Autodesk Inventor part; units mm, degrees
(part 2 of 3)
sketch "Sketch18" plane through (0, 4, 0) normal (0, 1, 0) x (1, 0, 0)
  line L0 (-39.5, -116.5) -> (-38, -116.5)
  line L1 (-38, -116.5) -> (-38, -108.5)
  line L2 (-38, -108.5) -> (-39.5, -108.5)
  line L3 (-39.5, -108.5) -> (-39.5, -116.5)
  line L4 (-40.75, -119.5) -> (-49.25, -119.5) projected
  line L5 (-40.75, -118) -> (-40.75, -119.5) projected
  line L6 (-24.5, -116.5) -> (-23, -116.5)
  line L7 (-23, -116.5) -> (-23, -108.5)
  line L8 (-23, -108.5) -> (-24.5, -108.5)
  line L9 (-24.5, -108.5) -> (-24.5, -116.5)
  line L10 (-9.5, -116.5) -> (-8, -116.5)
  line L11 (-8, -116.5) -> (-8, -108.5)
  line L12 (-8, -108.5) -> (-9.5, -108.5)
  line L13 (-9.5, -108.5) -> (-9.5, -116.5)
  line L14 (5.5, -116.5) -> (7, -116.5)
  line L15 (7, -116.5) -> (7, -108.5)
  line L16 (7, -108.5) -> (5.5, -108.5)
  line L17 (5.5, -108.5) -> (5.5, -116.5)
  line L18 (20.5, -116.5) -> (22, -116.5)
  line L19 (22, -116.5) -> (22, -108.5)
  line L20 (22, -108.5) -> (20.5, -108.5)
  line L21 (20.5, -108.5) -> (20.5, -116.5)
  line L22 (35.5, -116.5) -> (37, -116.5)
  line L23 (37, -116.5) -> (37, -108.5)
  line L24 (37, -108.5) -> (35.5, -108.5)
  line L25 (35.5, -108.5) -> (35.5, -116.5)
  line L26 (50.5, -116.5) -> (52, -116.5)
  line L27 (52, -116.5) -> (52, -108.5)
  line L28 (52, -108.5) -> (50.5, -108.5)
  line L29 (50.5, -108.5) -> (50.5, -116.5)
  line L30 (-39.5, -101.5) -> (-38, -101.5)
  line L31 (-38, -101.5) -> (-38, -93.5)
  line L32 (-38, -93.5) -> (-39.5, -93.5)
  line L33 (-39.5, -93.5) -> (-39.5, -101.5)
  line L34 (-24.5, -101.5) -> (-23, -101.5)
  line L35 (-23, -101.5) -> (-23, -93.5)
  line L36 (-23, -93.5) -> (-24.5, -93.5)
  line L37 (-24.5, -93.5) -> (-24.5, -101.5)
  line L38 (-9.5, -101.5) -> (-8, -101.5)
  line L39 (-8, -101.5) -> (-8, -93.5)
  line L40 (-8, -93.5) -> (-9.5, -93.5)
  line L41 (-9.5, -93.5) -> (-9.5, -101.5)
  line L42 (5.5, -101.5) -> (7, -101.5)
  line L43 (7, -101.5) -> (7, -93.5)
  line L44 (7, -93.5) -> (5.5, -93.5)
  line L45 (5.5, -93.5) -> (5.5, -101.5)
  line L46 (20.5, -101.5) -> (22, -101.5)
  line L47 (22, -101.5) -> (22, -93.5)
  line L48 (22, -93.5) -> (20.5, -93.5)
  line L49 (20.5, -93.5) -> (20.5, -101.5)
  line L50 (35.5, -101.5) -> (37, -101.5)
  line L51 (37, -101.5) -> (37, -93.5)
  line L52 (37, -93.5) -> (35.5, -93.5)
  line L53 (35.5, -93.5) -> (35.5, -101.5)
  line L54 (50.5, -101.5) -> (52, -101.5)
  line L55 (52, -101.5) -> (52, -93.5)
  line L56 (52, -93.5) -> (50.5, -93.5)
  line L57 (50.5, -93.5) -> (50.5, -101.5)
  line L58 (-39.5, -86.5) -> (-38, -86.5)
  line L59 (-38, -86.5) -> (-38, -78.5)
  line L60 (-38, -78.5) -> (-39.5, -78.5)
  line L61 (-39.5, -78.5) -> (-39.5, -86.5)
  line L62 (-24.5, -86.5) -> (-23, -86.5)
  line L63 (-23, -86.5) -> (-23, -78.5)
  line L64 (-23, -78.5) -> (-24.5, -78.5)
  line L65 (-24.5, -78.5) -> (-24.5, -86.5)
  line L66 (-9.5, -86.5) -> (-8, -86.5)
  line L67 (-8, -86.5) -> (-8, -78.5)
  line L68 (-8, -78.5) -> (-9.5, -78.5)
  line L69 (-9.5, -78.5) -> (-9.5, -86.5)
  line L70 (5.5, -86.5) -> (7, -86.5)
  line L71 (7, -86.5) -> (7, -78.5)
  line L72 (7, -78.5) -> (5.5, -78.5)
  line L73 (5.5, -78.5) -> (5.5, -86.5)
  line L74 (20.5, -86.5) -> (22, -86.5)
  line L75 (22, -86.5) -> (22, -78.5)
  line L76 (22, -78.5) -> (20.5, -78.5)
  line L77 (20.5, -78.5) -> (20.5, -86.5)
  line L78 (35.5, -86.5) -> (37, -86.5)
  line L79 (37, -86.5) -> (37, -78.5)
  line L80 (37, -78.5) -> (35.5, -78.5)
  line L81 (35.5, -78.5) -> (35.5, -86.5)
  line L82 (50.5, -86.5) -> (52, -86.5)
  line L83 (52, -86.5) -> (52, -78.5)
  line L84 (52, -78.5) -> (50.5, -78.5)
  line L85 (50.5, -78.5) -> (50.5, -86.5)
  line L86 (-39.5, -71.5) -> (-38, -71.5)
  line L87 (-38, -71.5) -> (-38, -63.5)
  line L88 (-38, -63.5) -> (-39.5, -63.5)
  line L89 (-39.5, -63.5) -> (-39.5, -71.5)
  line L90 (-24.5, -71.5) -> (-23, -71.5)
  line L91 (-23, -71.5) -> (-23, -63.5)
  line L92 (-23, -63.5) -> (-24.5, -63.5)
  line L93 (-24.5, -63.5) -> (-24.5, -71.5)
  line L94 (-9.5, -71.5) -> (-8, -71.5)
  line L95 (-8, -71.5) -> (-8, -63.5)
  line L96 (-8, -63.5) -> (-9.5, -63.5)
  line L97 (-9.5, -63.5) -> (-9.5, -71.5)
  line L98 (5.5, -71.5) -> (7, -71.5)
  line L99 (7, -71.5) -> (7, -63.5)
  line L100 (7, -63.5) -> (5.5, -63.5)
  line L101 (5.5, -63.5) -> (5.5, -71.5)
  line L102 (20.5, -71.5) -> (22, -71.5)
  line L103 (22, -71.5) -> (22, -63.5)
  line L104 (22, -63.5) -> (20.5, -63.5)
  line L105 (20.5, -63.5) -> (20.5, -71.5)
  line L106 (35.5, -71.5) -> (37, -71.5)
  line L107 (37, -71.5) -> (37, -63.5)
  line L108 (37, -63.5) -> (35.5, -63.5)
  line L109 (35.5, -63.5) -> (35.5, -71.5)
  line L110 (50.5, -71.5) -> (52, -71.5)
  line L111 (52, -71.5) -> (52, -63.5)
  line L112 (52, -63.5) -> (50.5, -63.5)
  line L113 (50.5, -63.5) -> (50.5, -71.5)
  line L114 (-39.5, -56.5) -> (-38, -56.5)
  line L115 (-38, -56.5) -> (-38, -48.5)
  line L116 (-38, -48.5) -> (-39.5, -48.5)
  line L117 (-39.5, -48.5) -> (-39.5, -56.5)
  line L118 (-24.5, -56.5) -> (-23, -56.5)
  line L119 (-23, -56.5) -> (-23, -48.5)
  line L120 (-23, -48.5) -> (-24.5, -48.5)
  line L121 (-24.5, -48.5) -> (-24.5, -56.5)
  line L122 (-9.5, -56.5) -> (-8, -56.5)
  line L123 (-8, -56.5) -> (-8, -48.5)
  line L124 (-8, -48.5) -> (-9.5, -48.5)
  line L125 (-9.5, -48.5) -> (-9.5, -56.5)
  line L126 (5.5, -56.5) -> (7, -56.5)
  line L127 (7, -56.5) -> (7, -48.5)
  line L128 (7, -48.5) -> (5.5, -48.5)
  line L129 (5.5, -48.5) -> (5.5, -56.5)
  line L130 (20.5, -56.5) -> (22, -56.5)
  line L131 (22, -56.5) -> (22, -48.5)
  line L132 (22, -48.5) -> (20.5, -48.5)
  line L133 (20.5, -48.5) -> (20.5, -56.5)
  line L134 (35.5, -56.5) -> (37, -56.5)
  line L135 (37, -56.5) -> (37, -48.5)
  line L136 (37, -48.5) -> (35.5, -48.5)
  line L137 (35.5, -48.5) -> (35.5, -56.5)
  line L138 (50.5, -56.5) -> (52, -56.5)
  line L139 (52, -56.5) -> (52, -48.5)
  line L140 (52, -48.5) -> (50.5, -48.5)
  line L141 (50.5, -48.5) -> (50.5, -56.5)
  line L142 (-39.5, -41.5) -> (-38, -41.5)
  line L143 (-38, -41.5) -> (-38, -33.5)
  line L144 (-38, -33.5) -> (-39.5, -33.5)
  line L145 (-39.5, -33.5) -> (-39.5, -41.5)
  line L146 (-24.5, -41.5) -> (-23, -41.5)
  line L147 (-23, -41.5) -> (-23, -33.5)
  line L148 (-23, -33.5) -> (-24.5, -33.5)
  line L149 (-24.5, -33.5) -> (-24.5, -41.5)
  line L150 (-9.5, -41.5) -> (-8, -41.5)
  line L151 (-8, -41.5) -> (-8, -33.5)
  line L152 (-8, -33.5) -> (-9.5, -33.5)
  line L153 (-9.5, -33.5) -> (-9.5, -41.5)
  line L154 (5.5, -41.5) -> (7, -41.5)
  line L155 (7, -41.5) -> (7, -33.5)
  line L156 (7, -33.5) -> (5.5, -33.5)
  line L157 (5.5, -33.5) -> (5.5, -41.5)
  line L158 (20.5, -41.5) -> (22, -41.5)
  line L159 (22, -41.5) -> (22, -33.5)
  line L160 (22, -33.5) -> (20.5, -33.5)
  line L161 (20.5, -33.5) -> (20.5, -41.5)
  line L162 (35.5, -41.5) -> (37, -41.5)
  line L163 (37, -41.5) -> (37, -33.5)
  line L164 (37, -33.5) -> (35.5, -33.5)
  line L165 (35.5, -33.5) -> (35.5, -41.5)
  line L166 (50.5, -41.5) -> (52, -41.5)
  line L167 (52, -41.5) -> (52, -33.5)
  line L168 (52, -33.5) -> (50.5, -33.5)
  line L169 (50.5, -33.5) -> (50.5, -41.5)
  line L170 (-39.5, -26.5) -> (-38, -26.5)
  line L171 (-38, -26.5) -> (-38, -18.5)
  line L172 (-38, -18.5) -> (-39.5, -18.5)
  line L173 (-39.5, -18.5) -> (-39.5, -26.5)
  line L174 (-24.5, -26.5) -> (-23, -26.5)
  line L175 (-23, -26.5) -> (-23, -18.5)
  line L176 (-23, -18.5) -> (-24.5, -18.5)
  line L177 (-24.5, -18.5) -> (-24.5, -26.5)
  line L178 (-9.5, -26.5) -> (-8, -26.5)
  line L179 (-8, -26.5) -> (-8, -18.5)
  line L180 (-8, -18.5) -> (-9.5, -18.5)
  line L181 (-9.5, -18.5) -> (-9.5, -26.5)
  line L182 (5.5, -26.5) -> (7, -26.5)
  line L183 (7, -26.5) -> (7, -18.5)
  line L184 (7, -18.5) -> (5.5, -18.5)
  line L185 (5.5, -18.5) -> (5.5, -26.5)
  line L186 (20.5, -26.5) -> (22, -26.5)
  line L187 (22, -26.5) -> (22, -18.5)
  line L188 (22, -18.5) -> (20.5, -18.5)
  line L189 (20.5, -18.5) -> (20.5, -26.5)
  line L190 (35.5, -26.5) -> (37, -26.5)
  line L191 (37, -26.5) -> (37, -18.5)
  line L192 (37, -18.5) -> (35.5, -18.5)
  line L193 (35.5, -18.5) -> (35.5, -26.5)
  line L194 (50.5, -26.5) -> (52, -26.5)
  line L195 (52, -26.5) -> (52, -18.5)
  line L196 (52, -18.5) -> (50.5, -18.5)
  line L197 (50.5, -18.5) -> (50.5, -26.5)
  line L198 (-39.5, -11.5) -> (-38, -11.5)
  line L199 (-38, -11.5) -> (-38, -3.5)
  line L200 (-38, -3.5) -> (-39.5, -3.5)
  line L201 (-39.5, -3.5) -> (-39.5, -11.5)
  line L202 (-24.5, -11.5) -> (-23, -11.5)
  line L203 (-23, -11.5) -> (-23, -3.5)
  line L204 (-23, -3.5) -> (-24.5, -3.5)
  line L205 (-24.5, -3.5) -> (-24.5, -11.5)
  line L206 (-9.5, -11.5) -> (-8, -11.5)
  line L207 (-8, -11.5) -> (-8, -3.5)
  line L208 (-8, -3.5) -> (-9.5, -3.5)
  line L209 (-9.5, -3.5) -> (-9.5, -11.5)
  line L210 (5.5, -11.5) -> (7, -11.5)
  line L211 (7, -11.5) -> (7, -3.5)
  line L212 (7, -3.5) -> (5.5, -3.5)
  line L213 (5.5, -3.5) -> (5.5, -11.5)
  line L214 (20.5, -11.5) -> (22, -11.5)
  line L215 (22, -11.5) -> (22, -3.5)
  line L216 (22, -3.5) -> (20.5, -3.5)
  line L217 (20.5, -3.5) -> (20.5, -11.5)
  line L218 (35.5, -11.5) -> (37, -11.5)
  line L219 (37, -11.5) -> (37, -3.5)
  line L220 (37, -3.5) -> (35.5, -3.5)
  line L221 (35.5, -3.5) -> (35.5, -11.5)
  line L222 (50.5, -11.5) -> (52, -11.5)
  line L223 (52, -11.5) -> (52, -3.5)
  line L224 (52, -3.5) -> (50.5, -3.5)
  line L225 (50.5, -3.5) -> (50.5, -11.5)
  line L226 (-39.5, 3.5) -> (-38, 3.5)
  line L227 (-38, 3.5) -> (-38, 11.5)
  line L228 (-38, 11.5) -> (-39.5, 11.5)
  line L229 (-39.5, 11.5) -> (-39.5, 3.5)
  line L230 (-24.5, 3.5) -> (-23, 3.5)
  line L231 (-23, 3.5) -> (-23, 11.5)
  line L232 (-23, 11.5) -> (-24.5, 11.5)
  line L233 (-24.5, 11.5) -> (-24.5, 3.5)
  line L234 (-9.5, 3.5) -> (-8, 3.5)
  line L235 (-8, 3.5) -> (-8, 11.5)
  line L236 (-8, 11.5) -> (-9.5, 11.5)
  line L237 (-9.5, 11.5) -> (-9.5, 3.5)
  line L238 (5.5, 3.5) -> (7, 3.5)
  line L239 (7, 3.5) -> (7, 11.5)
  line L240 (7, 11.5) -> (5.5, 11.5)
  line L241 (5.5, 11.5) -> (5.5, 3.5)
  line L242 (20.5, 3.5) -> (22, 3.5)
  line L243 (22, 3.5) -> (22, 11.5)
  line L244 (22, 11.5) -> (20.5, 11.5)
  line L245 (20.5, 11.5) -> (20.5, 3.5)
  line L246 (35.5, 3.5) -> (37, 3.5)
  line L247 (37, 3.5) -> (37, 11.5)
  line L248 (37, 11.5) -> (35.5, 11.5)
  line L249 (35.5, 11.5) -> (35.5, 3.5)
  line L250 (50.5, 3.5) -> (52, 3.5)
  line L251 (52, 3.5) -> (52, 11.5)
  line L252 (52, 11.5) -> (50.5, 11.5)
  line L253 (50.5, 11.5) -> (50.5, 3.5)
  line L254 (-39.5, 18.5) -> (-38, 18.5)
  line L255 (-38, 18.5) -> (-38, 26.5)
  line L256 (-38, 26.5) -> (-39.5, 26.5)
  line L257 (-39.5, 26.5) -> (-39.5, 18.5)
  line L258 (-24.5, 18.5) -> (-23, 18.5)
  line L259 (-23, 18.5) -> (-23, 26.5)
  line L260 (-23, 26.5) -> (-24.5, 26.5)
  line L261 (-24.5, 26.5) -> (-24.5, 18.5)
  line L262 (-9.5, 18.5) -> (-8, 18.5)
  line L263 (-8, 18.5) -> (-8, 26.5)
  line L264 (-8, 26.5) -> (-9.5, 26.5)
  line L265 (-9.5, 26.5) -> (-9.5, 18.5)
  line L266 (5.5, 18.5) -> (7, 18.5)
  line L267 (7, 18.5) -> (7, 26.5)
  line L268 (7, 26.5) -> (5.5, 26.5)
  line L269 (5.5, 26.5) -> (5.5, 18.5)
  line L270 (20.5, 18.5) -> (22, 18.5)
  line L271 (22, 18.5) -> (22, 26.5)
  line L272 (22, 26.5) -> (20.5, 26.5)
  line L273 (20.5, 26.5) -> (20.5, 18.5)
  line L274 (35.5, 18.5) -> (37, 18.5)
  line L275 (37, 18.5) -> (37, 26.5)
  line L276 (37, 26.5) -> (35.5, 26.5)
  line L277 (35.5, 26.5) -> (35.5, 18.5)
  line L278 (50.5, 18.5) -> (52, 18.5)
  line L279 (52, 18.5) -> (52, 26.5)
  line L280 (52, 26.5) -> (50.5, 26.5)
  line L281 (50.5, 26.5) -> (50.5, 18.5)
  line L282 (-39.5, 33.5) -> (-38, 33.5)
  line L283 (-38, 33.5) -> (-38, 41.5)
  line L284 (-38, 41.5) -> (-39.5, 41.5)
  line L285 (-39.5, 41.5) -> (-39.5, 33.5)
  line L286 (-24.5, 33.5) -> (-23, 33.5)
  line L287 (-23, 33.5) -> (-23, 41.5)
  line L288 (-23, 41.5) -> (-24.5, 41.5)
  line L289 (-24.5, 41.5) -> (-24.5, 33.5)
  line L290 (-9.5, 33.5) -> (-8, 33.5)
  line L291 (-8, 33.5) -> (-8, 41.5)
  line L292 (-8, 41.5) -> (-9.5, 41.5)
  line L293 (-9.5, 41.5) -> (-9.5, 33.5)
  line L294 (5.5, 33.5) -> (7, 33.5)
  line L295 (7, 33.5) -> (7, 41.5)
  line L296 (7, 41.5) -> (5.5, 41.5)
  line L297 (5.5, 41.5) -> (5.5, 33.5)
  line L298 (20.5, 33.5) -> (22, 33.5)
  line L299 (22, 33.5) -> (22, 41.5)
  line L300 (22, 41.5) -> (20.5, 41.5)
  line L301 (20.5, 41.5) -> (20.5, 33.5)
  line L302 (35.5, 33.5) -> (37, 33.5)
  line L303 (37, 33.5) -> (37, 41.5)
  line L304 (37, 41.5) -> (35.5, 41.5)
  line L305 (35.5, 41.5) -> (35.5, 33.5)
  line L306 (50.5, 33.5) -> (52, 33.5)
  line L307 (52, 33.5) -> (52, 41.5)
  line L308 (52, 41.5) -> (50.5, 41.5)
  line L309 (50.5, 41.5) -> (50.5, 33.5)
  line L310 (-39.5, 48.5) -> (-38, 48.5)
  line L311 (-38, 48.5) -> (-38, 56.5)
  line L312 (-38, 56.5) -> (-39.5, 56.5)
  line L313 (-39.5, 56.5) -> (-39.5, 48.5)
  line L314 (-24.5, 48.5) -> (-23, 48.5)
  line L315 (-23, 48.5) -> (-23, 56.5)
  line L316 (-23, 56.5) -> (-24.5, 56.5)
  line L317 (-24.5, 56.5) -> (-24.5, 48.5)
  line L318 (-9.5, 48.5) -> (-8, 48.5)
  line L319 (-8, 48.5) -> (-8, 56.5)
  line L320 (-8, 56.5) -> (-9.5, 56.5)
  line L321 (-9.5, 56.5) -> (-9.5, 48.5)
  line L322 (5.5, 48.5) -> (7, 48.5)
  line L323 (7, 48.5) -> (7, 56.5)
  line L324 (7, 56.5) -> (5.5, 56.5)
  line L325 (5.5, 56.5) -> (5.5, 48.5)
  line L326 (20.5, 48.5) -> (22, 48.5)
  line L327 (22, 48.5) -> (22, 56.5)
  line L328 (22, 56.5) -> (20.5, 56.5)
  line L329 (20.5, 56.5) -> (20.5, 48.5)
  line L330 (35.5, 48.5) -> (37, 48.5)
  line L331 (37, 48.5) -> (37, 56.5)
  line L332 (37, 56.5) -> (35.5, 56.5)
  line L333 (35.5, 56.5) -> (35.5, 48.5)
  line L334 (50.5, 48.5) -> (52, 48.5)
  line L335 (52, 48.5) -> (52, 56.5)
  line L336 (52, 56.5) -> (50.5, 56.5)
  line L337 (50.5, 56.5) -> (50.5, 48.5)
  line L338 (-39.5, 63.5) -> (-38, 63.5)
  line L339 (-38, 63.5) -> (-38, 71.5)
  line L340 (-38, 71.5) -> (-39.5, 71.5)
  line L341 (-39.5, 71.5) -> (-39.5, 63.5)
  line L342 (-24.5, 63.5) -> (-23, 63.5)
  line L343 (-23, 63.5) -> (-23, 71.5)
  line L344 (-23, 71.5) -> (-24.5, 71.5)
  line L345 (-24.5, 71.5) -> (-24.5, 63.5)
  line L346 (-9.5, 63.5) -> (-8, 63.5)
  line L347 (-8, 63.5) -> (-8, 71.5)
  line L348 (-8, 71.5) -> (-9.5, 71.5)
  line L349 (-9.5, 71.5) -> (-9.5, 63.5)
  line L350 (5.5, 63.5) -> (7, 63.5)
  line L351 (7, 63.5) -> (7, 71.5)
  line L352 (7, 71.5) -> (5.5, 71.5)
  line L353 (5.5, 71.5) -> (5.5, 63.5)
  line L354 (20.5, 63.5) -> (22, 63.5)
  line L355 (22, 63.5) -> (22, 71.5)
  line L356 (22, 71.5) -> (20.5, 71.5)
  line L357 (20.5, 71.5) -> (20.5, 63.5)
  line L358 (35.5, 63.5) -> (37, 63.5)
  line L359 (37, 63.5) -> (37, 71.5)
  line L360 (37, 71.5) -> (35.5, 71.5)
  line L361 (35.5, 71.5) -> (35.5, 63.5)
  line L362 (50.5, 63.5) -> (52, 63.5)
  line L363 (52, 63.5) -> (52, 71.5)
  line L364 (52, 71.5) -> (50.5, 71.5)
  line L365 (50.5, 71.5) -> (50.5, 63.5)
  line L366 (-39.5, 78.5) -> (-38, 78.5)
  line L367 (-38, 78.5) -> (-38, 86.5)
  line L368 (-38, 86.5) -> (-39.5, 86.5)
  line L369 (-39.5, 86.5) -> (-39.5, 78.5)
  line L370 (-24.5, 78.5) -> (-23, 78.5)
  line L371 (-23, 78.5) -> (-23, 86.5)
  line L372 (-23, 86.5) -> (-24.5, 86.5)
  line L373 (-24.5, 86.5) -> (-24.5, 78.5)
  line L374 (-9.5, 78.5) -> (-8, 78.5)
  line L375 (-8, 78.5) -> (-8, 86.5)
  line L376 (-8, 86.5) -> (-9.5, 86.5)
  line L377 (-9.5, 86.5) -> (-9.5, 78.5)
  line L378 (5.5, 78.5) -> (7, 78.5)
  line L379 (7, 78.5) -> (7, 86.5)
  line L380 (7, 86.5) -> (5.5, 86.5)
  line L381 (5.5, 86.5) -> (5.5, 78.5)
  line L382 (20.5, 78.5) -> (22, 78.5)
  line L383 (22, 78.5) -> (22, 86.5)
  line L384 (22, 86.5) -> (20.5, 86.5)
  line L385 (20.5, 86.5) -> (20.5, 78.5)
  line L386 (35.5, 78.5) -> (37, 78.5)
  line L387 (37, 78.5) -> (37, 86.5)
  line L388 (37, 86.5) -> (35.5, 86.5)
  line L389 (35.5, 86.5) -> (35.5, 78.5)
  line L390 (50.5, 78.5) -> (52, 78.5)
  line L391 (52, 78.5) -> (52, 86.5)
  line L392 (52, 86.5) -> (50.5, 86.5)
  line L393 (50.5, 86.5) -> (50.5, 78.5)
  line L394 (-39.5, 93.5) -> (-38, 93.5)
  line L395 (-38, 93.5) -> (-38, 101.5)
  line L396 (-38, 101.5) -> (-39.5, 101.5)
  line L397 (-39.5, 101.5) -> (-39.5, 93.5)
  line L398 (-24.5, 93.5) -> (-23, 93.5)
  line L399 (-23, 93.5) -> (-23, 101.5)
  line L400 (-23, 101.5) -> (-24.5, 101.5)
  line L401 (-24.5, 101.5) -> (-24.5, 93.5)
  line L402 (-9.5, 93.5) -> (-8, 93.5)
  line L403 (-8, 93.5) -> (-8, 101.5)
  line L404 (-8, 101.5) -> (-9.5, 101.5)
  line L405 (-9.5, 101.5) -> (-9.5, 93.5)
  line L406 (5.5, 93.5) -> (7, 93.5)
  line L407 (7, 93.5) -> (7, 101.5)
  line L408 (7, 101.5) -> (5.5, 101.5)
  line L409 (5.5, 101.5) -> (5.5, 93.5)
  line L410 (20.5, 93.5) -> (22, 93.5)
  line L411 (22, 93.5) -> (22, 101.5)
  line L412 (22, 101.5) -> (20.5, 101.5)
  line L413 (20.5, 101.5) -> (20.5, 93.5)
  line L414 (35.5, 93.5) -> (37, 93.5)
  line L415 (37, 93.5) -> (37, 101.5)
  line L416 (37, 101.5) -> (35.5, 101.5)
  line L417 (35.5, 101.5) -> (35.5, 93.5)
  line L418 (50.5, 93.5) -> (52, 93.5)
  line L419 (52, 93.5) -> (52, 101.5)
  line L420 (52, 101.5) -> (50.5, 101.5)
  line L421 (50.5, 101.5) -> (50.5, 93.5)
  line L422 (-39.5, 108.5) -> (-38, 108.5)
  line L423 (-38, 108.5) -> (-38, 116.5)
  line L424 (-38, 116.5) -> (-39.5, 116.5)
  line L425 (-39.5, 116.5) -> (-39.5, 108.5)
  line L426 (-24.5, 108.5) -> (-23, 108.5)
  line L427 (-23, 108.5) -> (-23, 116.5)
  line L428 (-23, 116.5) -> (-24.5, 116.5)
  line L429 (-24.5, 116.5) -> (-24.5, 108.5)
  line L430 (-9.5, 108.5) -> (-8, 108.5)
  line L431 (-8, 108.5) -> (-8, 116.5)
  line L432 (-8, 116.5) -> (-9.5, 116.5)
  line L433 (-9.5, 116.5) -> (-9.5, 108.5)
  line L434 (5.5, 108.5) -> (7, 108.5)
  line L435 (7, 108.5) -> (7, 116.5)
  line L436 (7, 116.5) -> (5.5, 116.5)
  line L437 (5.5, 116.5) -> (5.5, 108.5)
  line L438 (20.5, 108.5) -> (22, 108.5)
  line L439 (22, 108.5) -> (22, 116.5)
  line L440 (22, 116.5) -> (20.5, 116.5)
  line L441 (20.5, 116.5) -> (20.5, 108.5)
  line L442 (35.5, 108.5) -> (37, 108.5)
  line L443 (37, 108.5) -> (37, 116.5)
  line L444 (37, 116.5) -> (35.5, 116.5)
  line L445 (35.5, 116.5) -> (35.5, 108.5)
  line L446 (50.5, 108.5) -> (52, 108.5)
  line L447 (52, 108.5) -> (52, 116.5)
  line L448 (52, 116.5) -> (50.5, 116.5)
  line L449 (50.5, 116.5) -> (50.5, 108.5)
  line L450 (19.25, -89.5) -> (10.75, -89.5) projected
  line L451 (20.5, -82.75) -> (22, -82.75)
  line L452 (22, -82.75) -> (22, -74.75)
  line L453 (22, -74.75) -> (20.5, -74.75)
  line L454 (20.5, -74.75) -> (20.5, -82.75)
  line L455 (20.5, -60.25) -> (22, -60.25)
  line L456 (22, -60.25) -> (22, -52.25)
  line L457 (22, -52.25) -> (20.5, -52.25)
  line L458 (20.5, -52.25) -> (20.5, -60.25)
  line L459 (20.5, -37.75) -> (22, -37.75)
  line L460 (22, -37.75) -> (22, -29.75)
  line L461 (22, -29.75) -> (20.5, -29.75)
  line L462 (20.5, -29.75) -> (20.5, -37.75)
  line L463 (19.25, -44.5) -> (10.75, -44.5) projected
  line L464 (20.5, -19) -> (22, -19)
  line L465 (22, -19) -> (22, -11)
  line L466 (22, -11) -> (20.5, -11)
  line L467 (20.5, -11) -> (20.5, -19)
  line L468 (10.75, -20.5) -> (19.25, -20.5) projected
  line L469 (19.25, -22) -> (10.75, -22) projected
  line L470 (19.25, -8) -> (19.25, -9.5) projected
  line L471 (20.5, -0.25) -> (22, -0.25)
  line L472 (22, -0.25) -> (22, 7.75)
  line L473 (22, 7.75) -> (20.5, 7.75)
  line L474 (20.5, 7.75) -> (20.5, -0.25)
  line L475 (20.5, 22.25) -> (22, 22.25)
  line L476 (22, 22.25) -> (22, 30.25)
  line L477 (22, 30.25) -> (20.5, 30.25)
  line L478 (20.5, 30.25) -> (20.5, 22.25)
  line L479 (20.5, 44.75) -> (22, 44.75)
  line L480 (22, 44.75) -> (22, 52.75)
  line L481 (22, 52.75) -> (20.5, 52.75)
  line L482 (20.5, 52.75) -> (20.5, 44.75)
  line L483 (20.5, 67.25) -> (22, 67.25)
  line L484 (22, 67.25) -> (22, 75.25)
  line L485 (22, 75.25) -> (20.5, 75.25)
  line L486 (20.5, 75.25) -> (20.5, 67.25)
  line L487 (20.5, 86) -> (22, 86)
  line L488 (22, 86) -> (22, 94)
  line L489 (22, 94) -> (20.5, 94)
  line L490 (20.5, 94) -> (20.5, 86)
  line L491 (20.5, 104.75) -> (22, 104.75)
  line L492 (22, 104.75) -> (22, 112.75)
  line L493 (22, 112.75) -> (20.5, 112.75)
  line L494 (20.5, 112.75) -> (20.5, 104.75)
  line L495 (19.25, 83) -> (10.75, 83) projected
  line L496 (19.25, 60.5) -> (10.75, 60.5) projected
  line L497 (10.75, 59.5) -> (19.25, 59.5) projected
  line L498 (10.75, 14.5) -> (19.25, 14.5) projected
  line L499 (10.75, -45.5) -> (19.25, -45.5) projected
  line L500 (19.25, 98) -> (10.75, 98) projected
  line L501 (10.75, 37) -> (19.25, 37) projected
  point P0 (0, 0)
  point P1 (20.5, -81.75)
  point P2 (20.5, -63)
  point P3 (22, -55)
  point P4 (20.5, -36.25)
  point P5 (20.5, -21.75)
  point P6 (20.25, -7)
  point P7 (20.5, 8.75)
  point P8 (22, 0.75)
  point P9 (20.5, 23.25)
  point P10 (22, 31.25)
  point P11 (20.5, 42)
  point P12 (22, 50)
  point P13 (20.5, 68.75)
  point P14 (22, 60.75)
  point P15 (20.5, 83.25)
  point P16 (22, 113.75)
  point P17 (20.5, 112.75)
  point P18 (20.5, 108.5)
  point P19 (22, 108.5)
  point P20 (20.5, 86)
  point P21 (22, 86)
  point P22 (22, 86.5)
  point P23 (22, 93.5)
  point P24 (22, 94)
  point P25 (20.5, 94)
  point P26 (20.5, 93.5)
  point P27 (20.5, 86.5)
  point P28 (22, 67.25)
  point P29 (22, 71.5)
  point P30 (20.5, 71.5)
  point P31 (20.5, 52.75)
  point P32 (20.5, 48.5)
  point P33 (22, 48.5)
  point P34 (22, 22.25)
  point P35 (22, 26.5)
  point P36 (20.5, 26.5)
  point P37 (20.5, 7.75)
  point P38 (20.5, 3.5)
  point P39 (22, 3.5)
  point P40 (20.5, -19)
  point P41 (22, -19)
  point P42 (22, -18.5)
  point P43 (22, -11.5)
  point P44 (22, -11)
  point P45 (20.5, -11)
  point P46 (20.5, -11.5)
  point P47 (20.5, -18.5)
  point P48 (22, -37.75)
  point P49 (22, -33.5)
  point P50 (20.5, -33.5)
  point P51 (20.5, -52.25)
  point P52 (20.5, -56.5)
  point P53 (22, -56.5)
  point P54 (22, -82.75)
  point P55 (22, -78.5)
  point P56 (20.5, -78.5)
  dimension "d177" = 8
  dimension "d178" = 1.5
  dimension "d179" = 3
  dimension "d180" = 1.25
  dimension "d187" = 15
  dimension "d190" = 15
  dimension "d296" = 6.75
  dimension "d297" = 8
  dimension "d298" = 1.5
  dimension "d300" = 8
  dimension "d301" = 6.75
  dimension "d302" = 8
  dimension "d303" = 1.5
  dimension "d304" = 8
  dimension "d306" = 3
  dimension "d307" = 1.5
  dimension "d308" = 1.25
  dimension "d309" = 8
  dimension "d310" = 8
  dimension "d311" = 8
  dimension "d312" = 8
  dimension "d313" = 8
  dimension "d314" = 8
  dimension "d316" = 3
  dimension "d317" = 6.75
  dimension "d318" = 6.75
  dimension "d320" = 6.75
  dimension "d321" = 1.5
  dimension "d323" = 6.75
  dimension "d324" = 6.75
  dimension "d325" = 6.75
  constraints: 976 end point, 30 point on line, 22 parallel, 12 horizontal, 11 perpendicular, 1 vertical, 889 other
  measures "d177" distance of L2.end L0.start
  measures "d178" distance of L1.end L2.end
  measures "d179" distance between parallel lines of L4 L0
  measures "d180" distance between parallel lines of L5 L3
  measures "d187" distance of L0.start L6.start
  measures "d190" distance of L0.start L30.start
  measures "d296" distance between parallel lines of L450 L451
  measures "d297" distance of L451.end L452.end
  measures "d298" distance of L452.end L453.end
  measures "d300" distance of L455.end L456.end
  measures "d301" distance between parallel lines of L463 L459
  measures "d302" distance of L459.end L460.end
  measures "d303" distance of L460.end L461.end
  measures "d304" distance of L464.end L465.end
  measures "d306" distance between parallel lines of L469 L464
  measures "d307" distance of L465.end L466.end
  measures "d309" distance of L471.end L472.end
  measures "d310" distance of L475.end L476.end
  measures "d311" distance of L479.end L480.end
  measures "d312" distance of L483.end L484.end
  measures "d313" distance of L487.end L488.end
  measures "d314" distance of L491.end L492.end
  measures "d316" distance between parallel lines of L495 L487
  measures "d317" distance between parallel lines of L496 L483
  measures "d318" distance between parallel lines of L497 L481
  measures "d320" distance between parallel lines of L498 L473
  measures "d321" distance of L471.start L471.end
  measures "d323" distance between parallel lines of L499 L457
  measures "d324" distance between parallel lines of L500 L491
  measures "d325" distance between parallel lines of L501 L477
extrude "Extrusion7" cut sketch "Sketch18" against normal blind 8 contours L3 L2 L1 L0 | L9 L8 L7 L6 | L13 L12 L11 L10 | L17 L16 L15 L14 | L21 L20 L19 L18 | L25 L24 L23 L22 | L29 L28 L27 L26 | L33 L32 L31 L30 | L37 L36 L35 L34 | L41 L40 L39 L38 | L45 L44 L43 L42 | L49 L48 L47 L46 | L53 L52 L51 L50 | L57 L56 L55 L54 | L77 L76 L75 L451 | L454 L453 L452 L76 | L85 L84 L83 L82 | L113 L112 L111 L110 | L133 L457 L131 L130 | L130 L456 L455 L458 | L141 L140 L139 L138 | L161 L160 L159 L459 | L462 L461 L460 L160 | L169 L168 L167 L166 | L189 L188 L187 L464 | L467 L214 L465 L188 | L217 L466 L215 L214 | L197 L196 L195 L194 | L225 L224 L223 L222 | L237 L236 L235 L234 | L241 L240 L239 L238 | L245 L473 L243 L242 | L242 L472 L471 L474 | L253 L252 L251 L250 | L265 L264 L263 L262 | L269 L268 L267 L266 | L273 L272 L271 L475 | L478 L477 L476 L272 | L281 L280 L279 L278 | L293 L292 L291 L290 | L297 L296 L295 L294 | L309 L308 L307 L306 | L321 L320 L319 L318 | L325 L324 L323 L322 | L329 L481 L327 L326 | L326 L480 L479 L482 | L337 L336 L335 L334 | L349 L348 L347 L346 | L353 L352 L351 L350 | L357 L356 L355 L483 | L486 L485 L484 L356 | L365 L364 L363 L362 | L377 L376 L375 L374 | L381 L380 L379 L378 | L385 L384 L383 L487 | L490 L410 L488 L384 | L413 L489 L411 L410 | L393 L392 L391 L390 | L405 L404 L403 L402 | L409 L408 L407 L406 | L421 L420 L419 L418 | L433 L432 L431 L430 | L437 L436 L435 L434 | L441 L493 L439 L438 | L438 L492 L491 L494 | L449 L448 L447 L446
sketch "Sketch21" plane through (0, 4, 0) normal (0, 1, 0) x (1, 0, 0)
  line L0 (-39.75, -117.75) -> (-50.25, -117.75)
  line L1 (-50.25, -117.75) -> (-50.25, -107.25)
  line L2 (-50.25, -107.25) -> (-39.75, -107.25)
  line L3 (-39.75, -107.25) -> (-39.75, -117.75)
  line L4 (-49.25, -118) -> (-40.75, -118) projected
  line L5 (-39.5, -116.5) -> (-39.5, -108.5) projected
  line L6 (-39.75, -102.75) -> (-50.25, -102.75)
  line L7 (-50.25, -102.75) -> (-50.25, -92.25)
  line L8 (-50.25, -92.25) -> (-39.75, -92.25)
  line L9 (-39.75, -92.25) -> (-39.75, -102.75)
  line L10 (-39.75, -87.75) -> (-50.25, -87.75)
  line L11 (-50.25, -87.75) -> (-50.25, -77.25)
  line L12 (-50.25, -77.25) -> (-39.75, -77.25)
  line L13 (-39.75, -77.25) -> (-39.75, -87.75)
  line L14 (-39.75, -72.75) -> (-50.25, -72.75)
  line L15 (-50.25, -72.75) -> (-50.25, -62.25)
  line L16 (-50.25, -62.25) -> (-39.75, -62.25)
  line L17 (-39.75, -62.25) -> (-39.75, -72.75)
  line L18 (-39.75, -57.75) -> (-50.25, -57.75)
  line L19 (-50.25, -57.75) -> (-50.25, -47.25)
  line L20 (-50.25, -47.25) -> (-39.75, -47.25)
  line L21 (-39.75, -47.25) -> (-39.75, -57.75)
  line L22 (-39.75, -42.75) -> (-50.25, -42.75)
  line L23 (-50.25, -42.75) -> (-50.25, -32.25)
  line L24 (-50.25, -32.25) -> (-39.75, -32.25)
  line L25 (-39.75, -32.25) -> (-39.75, -42.75)
  line L26 (-39.75, -27.75) -> (-50.25, -27.75)
  line L27 (-50.25, -27.75) -> (-50.25, -17.25)
  line L28 (-50.25, -17.25) -> (-39.75, -17.25)
  line L29 (-39.75, -17.25) -> (-39.75, -27.75)
  line L30 (-39.75, -12.75) -> (-50.25, -12.75)
  line L31 (-50.25, -12.75) -> (-50.25, -2.25)
  line L32 (-50.25, -2.25) -> (-39.75, -2.25)
  line L33 (-39.75, -2.25) -> (-39.75, -12.75)
  line L34 (-39.75, 2.25) -> (-50.25, 2.25)
  line L35 (-50.25, 2.25) -> (-50.25, 12.75)
  line L36 (-50.25, 12.75) -> (-39.75, 12.75)
  line L37 (-39.75, 12.75) -> (-39.75, 2.25)
  line L38 (-39.75, 17.25) -> (-50.25, 17.25)
  line L39 (-50.25, 17.25) -> (-50.25, 27.75)
  line L40 (-50.25, 27.75) -> (-39.75, 27.75)
  line L41 (-39.75, 27.75) -> (-39.75, 17.25)
  line L42 (-39.75, 32.25) -> (-50.25, 32.25)
  line L43 (-50.25, 32.25) -> (-50.25, 42.75)
  line L44 (-50.25, 42.75) -> (-39.75, 42.75)
  line L45 (-39.75, 42.75) -> (-39.75, 32.25)
  line L46 (-39.75, 47.25) -> (-50.25, 47.25)
  line L47 (-50.25, 47.25) -> (-50.25, 57.75)
  line L48 (-50.25, 57.75) -> (-39.75, 57.75)
  line L49 (-39.75, 57.75) -> (-39.75, 47.25)
  line L50 (-39.75, 62.25) -> (-50.25, 62.25)
  line L51 (-50.25, 62.25) -> (-50.25, 72.75)
  line L52 (-50.25, 72.75) -> (-39.75, 72.75)
  line L53 (-39.75, 72.75) -> (-39.75, 62.25)
  line L54 (-39.75, 77.25) -> (-50.25, 77.25)
  line L55 (-50.25, 77.25) -> (-50.25, 87.75)
  line L56 (-50.25, 87.75) -> (-39.75, 87.75)
  line L57 (-39.75, 87.75) -> (-39.75, 77.25)
  line L58 (-39.75, 92.25) -> (-50.25, 92.25)
  line L59 (-50.25, 92.25) -> (-50.25, 102.75)
  line L60 (-50.25, 102.75) -> (-39.75, 102.75)
  line L61 (-39.75, 102.75) -> (-39.75, 92.25)
  line L62 (-39.75, 107.25) -> (-50.25, 107.25)
  line L63 (-50.25, 107.25) -> (-50.25, 117.75)
  line L64 (-50.25, 117.75) -> (-39.75, 117.75)
  line L65 (-39.75, 117.75) -> (-39.75, 107.25)
  line L66 (-24.75, -117.75) -> (-35.25, -117.75)
  line L67 (-35.25, -117.75) -> (-35.25, -107.25)
  line L68 (-35.25, -107.25) -> (-24.75, -107.25)
  line L69 (-24.75, -107.25) -> (-24.75, -117.75)
  line L70 (-24.75, -102.75) -> (-35.25, -102.75)
  line L71 (-35.25, -102.75) -> (-35.25, -92.25)
  line L72 (-35.25, -92.25) -> (-24.75, -92.25)
  line L73 (-24.75, -92.25) -> (-24.75, -102.75)
  line L74 (-24.75, -87.75) -> (-35.25, -87.75)
  line L75 (-35.25, -87.75) -> (-35.25, -77.25)
  line L76 (-35.25, -77.25) -> (-24.75, -77.25)
  line L77 (-24.75, -77.25) -> (-24.75, -87.75)
  line L78 (-24.75, -72.75) -> (-35.25, -72.75)
  line L79 (-35.25, -72.75) -> (-35.25, -62.25)
  line L80 (-35.25, -62.25) -> (-24.75, -62.25)
  line L81 (-24.75, -62.25) -> (-24.75, -72.75)
  line L82 (-24.75, -57.75) -> (-35.25, -57.75)
  line L83 (-35.25, -57.75) -> (-35.25, -47.25)
  line L84 (-35.25, -47.25) -> (-24.75, -47.25)
  line L85 (-24.75, -47.25) -> (-24.75, -57.75)
  line L86 (-24.75, -42.75) -> (-35.25, -42.75)
  line L87 (-35.25, -42.75) -> (-35.25, -32.25)
  line L88 (-35.25, -32.25) -> (-24.75, -32.25)
  line L89 (-24.75, -32.25) -> (-24.75, -42.75)
  line L90 (-24.75, -27.75) -> (-35.25, -27.75)
  line L91 (-35.25, -27.75) -> (-35.25, -17.25)
  line L92 (-35.25, -17.25) -> (-24.75, -17.25)
  line L93 (-24.75, -17.25) -> (-24.75, -27.75)
  line L94 (-24.75, -12.75) -> (-35.25, -12.75)
  line L95 (-35.25, -12.75) -> (-35.25, -2.25)
  line L96 (-35.25, -2.25) -> (-24.75, -2.25)
  line L97 (-24.75, -2.25) -> (-24.75, -12.75)
  line L98 (-24.75, 2.25) -> (-35.25, 2.25)
  line L99 (-35.25, 2.25) -> (-35.25, 12.75)
  line L100 (-35.25, 12.75) -> (-24.75, 12.75)
  line L101 (-24.75, 12.75) -> (-24.75, 2.25)
  line L102 (-24.75, 17.25) -> (-35.25, 17.25)
  line L103 (-35.25, 17.25) -> (-35.25, 27.75)
  line L104 (-35.25, 27.75) -> (-24.75, 27.75)
  line L105 (-24.75, 27.75) -> (-24.75, 17.25)
  line L106 (-24.75, 32.25) -> (-35.25, 32.25)
  line L107 (-35.25, 32.25) -> (-35.25, 42.75)
  line L108 (-35.25, 42.75) -> (-24.75, 42.75)
  line L109 (-24.75, 42.75) -> (-24.75, 32.25)
  line L110 (-24.75, 47.25) -> (-35.25, 47.25)
  line L111 (-35.25, 47.25) -> (-35.25, 57.75)
  line L112 (-35.25, 57.75) -> (-24.75, 57.75)
  line L113 (-24.75, 57.75) -> (-24.75, 47.25)
  line L114 (-24.75, 62.25) -> (-35.25, 62.25)
  line L115 (-35.25, 62.25) -> (-35.25, 72.75)
  line L116 (-35.25, 72.75) -> (-24.75, 72.75)
  line L117 (-24.75, 72.75) -> (-24.75, 62.25)
  line L118 (-24.75, 77.25) -> (-35.25, 77.25)
  line L119 (-35.25, 77.25) -> (-35.25, 87.75)
  line L120 (-35.25, 87.75) -> (-24.75, 87.75)
  line L121 (-24.75, 87.75) -> (-24.75, 77.25)
  line L122 (-24.75, 92.25) -> (-35.25, 92.25)
  line L123 (-35.25, 92.25) -> (-35.25, 102.75)
  line L124 (-35.25, 102.75) -> (-24.75, 102.75)
  line L125 (-24.75, 102.75) -> (-24.75, 92.25)
  line L126 (-24.75, 107.25) -> (-35.25, 107.25)
  line L127 (-35.25, 107.25) -> (-35.25, 117.75)
  line L128 (-35.25, 117.75) -> (-24.75, 117.75)
  line L129 (-24.75, 117.75) -> (-24.75, 107.25)
  line L130 (-9.75, -117.75) -> (-20.25, -117.75)
  line L131 (-20.25, -117.75) -> (-20.25, -107.25)
  line L132 (-20.25, -107.25) -> (-9.75, -107.25)
  line L133 (-9.75, -107.25) -> (-9.75, -117.75)
  line L134 (-9.75, -102.75) -> (-20.25, -102.75)
  line L135 (-20.25, -102.75) -> (-20.25, -92.25)
  line L136 (-20.25, -92.25) -> (-9.75, -92.25)
  line L137 (-9.75, -92.25) -> (-9.75, -102.75)
  line L138 (-9.75, -87.75) -> (-20.25, -87.75)
  line L139 (-20.25, -87.75) -> (-20.25, -77.25)
  line L140 (-20.25, -77.25) -> (-9.75, -77.25)
  line L141 (-9.75, -77.25) -> (-9.75, -87.75)
  line L142 (-9.75, -72.75) -> (-20.25, -72.75)
  line L143 (-20.25, -72.75) -> (-20.25, -62.25)
  line L144 (-20.25, -62.25) -> (-9.75, -62.25)
  line L145 (-9.75, -62.25) -> (-9.75, -72.75)
  line L146 (-9.75, -57.75) -> (-20.25, -57.75)
  line L147 (-20.25, -57.75) -> (-20.25, -47.25)
  line L148 (-20.25, -47.25) -> (-9.75, -47.25)
  line L149 (-9.75, -47.25) -> (-9.75, -57.75)
  line L150 (-9.75, -42.75) -> (-20.25, -42.75)
  line L151 (-20.25, -42.75) -> (-20.25, -32.25)
  line L152 (-20.25, -32.25) -> (-9.75, -32.25)
  line L153 (-9.75, -32.25) -> (-9.75, -42.75)
  line L154 (-9.75, -27.75) -> (-20.25, -27.75)
  line L155 (-20.25, -27.75) -> (-20.25, -17.25)
  line L156 (-20.25, -17.25) -> (-9.75, -17.25)
  line L157 (-9.75, -17.25) -> (-9.75, -27.75)
  line L158 (-9.75, -12.75) -> (-20.25, -12.75)
  line L159 (-20.25, -12.75) -> (-20.25, -2.25)
  line L160 (-20.25, -2.25) -> (-9.75, -2.25)
  line L161 (-9.75, -2.25) -> (-9.75, -12.75)
  line L162 (-9.75, 2.25) -> (-20.25, 2.25)
  line L163 (-20.25, 2.25) -> (-20.25, 12.75)
  line L164 (-20.25, 12.75) -> (-9.75, 12.75)
  line L165 (-9.75, 12.75) -> (-9.75, 2.25)
  line L166 (-9.75, 17.25) -> (-20.25, 17.25)
  line L167 (-20.25, 17.25) -> (-20.25, 27.75)
  line L168 (-20.25, 27.75) -> (-9.75, 27.75)
  line L169 (-9.75, 27.75) -> (-9.75, 17.25)
  line L170 (-9.75, 32.25) -> (-20.25, 32.25)
  line L171 (-20.25, 32.25) -> (-20.25, 42.75)
  line L172 (-20.25, 42.75) -> (-9.75, 42.75)
  line L173 (-9.75, 42.75) -> (-9.75, 32.25)
  line L174 (-9.75, 47.25) -> (-20.25, 47.25)
  line L175 (-20.25, 47.25) -> (-20.25, 57.75)
  line L176 (-20.25, 57.75) -> (-9.75, 57.75)
  line L177 (-9.75, 57.75) -> (-9.75, 47.25)
  line L178 (-9.75, 62.25) -> (-20.25, 62.25)
  line L179 (-20.25, 62.25) -> (-20.25, 72.75)
  line L180 (-20.25, 72.75) -> (-9.75, 72.75)
  line L181 (-9.75, 72.75) -> (-9.75, 62.25)
  line L182 (-9.75, 77.25) -> (-20.25, 77.25)
  line L183 (-20.25, 77.25) -> (-20.25, 87.75)
  line L184 (-20.25, 87.75) -> (-9.75, 87.75)
  line L185 (-9.75, 87.75) -> (-9.75, 77.25)
  line L186 (-9.75, 92.25) -> (-20.25, 92.25)
  line L187 (-20.25, 92.25) -> (-20.25, 102.75)
  line L188 (-20.25, 102.75) -> (-9.75, 102.75)
  line L189 (-9.75, 102.75) -> (-9.75, 92.25)
  line L190 (-9.75, 107.25) -> (-20.25, 107.25)
  line L191 (-20.25, 107.25) -> (-20.25, 117.75)
  line L192 (-20.25, 117.75) -> (-9.75, 117.75)
  line L193 (-9.75, 117.75) -> (-9.75, 107.25)
  line L194 (5.25, -117.75) -> (-5.25, -117.75)
  line L195 (-5.25, -117.75) -> (-5.25, -107.25)
  line L196 (-5.25, -107.25) -> (5.25, -107.25)
  line L197 (5.25, -107.25) -> (5.25, -117.75)
  line L198 (5.25, -102.75) -> (-5.25, -102.75)
  line L199 (-5.25, -102.75) -> (-5.25, -92.25)
  line L200 (-5.25, -92.25) -> (5.25, -92.25)
  line L201 (5.25, -92.25) -> (5.25, -102.75)
  line L202 (5.25, -87.75) -> (-5.25, -87.75)
  line L203 (-5.25, -87.75) -> (-5.25, -77.25)
  line L204 (-5.25, -77.25) -> (5.25, -77.25)
  line L205 (5.25, -77.25) -> (5.25, -87.75)
  line L206 (5.25, -72.75) -> (-5.25, -72.75)
  line L207 (-5.25, -72.75) -> (-5.25, -62.25)
  line L208 (-5.25, -62.25) -> (5.25, -62.25)
  line L209 (5.25, -62.25) -> (5.25, -72.75)
  line L210 (5.25, -57.75) -> (-5.25, -57.75)
  line L211 (-5.25, -57.75) -> (-5.25, -47.25)
  line L212 (-5.25, -47.25) -> (5.25, -47.25)
  line L213 (5.25, -47.25) -> (5.25, -57.75)
  line L214 (5.25, -42.75) -> (-5.25, -42.75)
  line L215 (-5.25, -42.75) -> (-5.25, -32.25)
  line L216 (-5.25, -32.25) -> (5.25, -32.25)
  line L217 (5.25, -32.25) -> (5.25, -42.75)
  line L218 (5.25, -27.75) -> (-5.25, -27.75)
  line L219 (-5.25, -27.75) -> (-5.25, -17.25)
  line L220 (-5.25, -17.25) -> (5.25, -17.25)
  line L221 (5.25, -17.25) -> (5.25, -27.75)
  line L222 (5.25, -12.75) -> (-5.25, -12.75)
  line L223 (-5.25, -12.75) -> (-5.25, -2.25)
  line L224 (-5.25, -2.25) -> (5.25, -2.25)
  line L225 (5.25, -2.25) -> (5.25, -12.75)
  line L226 (5.25, 2.25) -> (-5.25, 2.25)
  line L227 (-5.25, 2.25) -> (-5.25, 12.75)
  line L228 (-5.25, 12.75) -> (5.25, 12.75)
  line L229 (5.25, 12.75) -> (5.25, 2.25)
  line L230 (5.25, 17.25) -> (-5.25, 17.25)
  line L231 (-5.25, 17.25) -> (-5.25, 27.75)
  line L232 (-5.25, 27.75) -> (5.25, 27.75)
  line L233 (5.25, 27.75) -> (5.25, 17.25)
  line L234 (5.25, 32.25) -> (-5.25, 32.25)
  line L235 (-5.25, 32.25) -> (-5.25, 42.75)
  line L236 (-5.25, 42.75) -> (5.25, 42.75)
  line L237 (5.25, 42.75) -> (5.25, 32.25)
  line L238 (5.25, 47.25) -> (-5.25, 47.25)
  line L239 (-5.25, 47.25) -> (-5.25, 57.75)
  line L240 (-5.25, 57.75) -> (5.25, 57.75)
  line L241 (5.25, 57.75) -> (5.25, 47.25)
  line L242 (5.25, 62.25) -> (-5.25, 62.25)
  line L243 (-5.25, 62.25) -> (-5.25, 72.75)
  line L244 (-5.25, 72.75) -> (5.25, 72.75)
  line L245 (5.25, 72.75) -> (5.25, 62.25)
  line L246 (5.25, 77.25) -> (-5.25, 77.25)
  line L247 (-5.25, 77.25) -> (-5.25, 87.75)
  line L248 (-5.25, 87.75) -> (5.25, 87.75)
  line L249 (5.25, 87.75) -> (5.25, 77.25)
  line L250 (5.25, 92.25) -> (-5.25, 92.25)
  line L251 (-5.25, 92.25) -> (-5.25, 102.75)
  line L252 (-5.25, 102.75) -> (5.25, 102.75)
  line L253 (5.25, 102.75) -> (5.25, 92.25)
  line L254 (5.25, 107.25) -> (-5.25, 107.25)
  line L255 (-5.25, 107.25) -> (-5.25, 117.75)
  line L256 (-5.25, 117.75) -> (5.25, 117.75)
  line L257 (5.25, 117.75) -> (5.25, 107.25)
  line L258 (20.25, -117.75) -> (9.75, -117.75)
  line L259 (9.75, -117.75) -> (9.75, -107.25)
  line L260 (9.75, -107.25) -> (20.25, -107.25)
  line L261 (20.25, -107.25) -> (20.25, -117.75)
  line L262 (20.25, -102.75) -> (9.75, -102.75)
  line L263 (9.75, -102.75) -> (9.75, -92.25)
  line L264 (9.75, -92.25) -> (20.25, -92.25)
  line L265 (20.25, -92.25) -> (20.25, -102.75)
  line L266 (20.25, -87.75) -> (9.75, -87.75)
  line L267 (9.75, -87.75) -> (9.75, -77.25)
  line L268 (9.75, -77.25) -> (20.25, -77.25)
  line L269 (20.25, -77.25) -> (20.25, -87.75)
  line L270 (20.25, -72.75) -> (9.75, -72.75)
  line L271 (9.75, -72.75) -> (9.75, -62.25)
  line L272 (9.75, -62.25) -> (20.25, -62.25)
  line L273 (20.25, -62.25) -> (20.25, -72.75)
  line L274 (20.25, -57.75) -> (9.75, -57.75)
  line L275 (9.75, -57.75) -> (9.75, -47.25)
  line L276 (9.75, -47.25) -> (20.25, -47.25)
  line L277 (20.25, -47.25) -> (20.25, -57.75)
  line L278 (20.25, -42.75) -> (9.75, -42.75)
  line L279 (9.75, -42.75) -> (9.75, -32.25)
  line L280 (9.75, -32.25) -> (20.25, -32.25)
  line L281 (20.25, -32.25) -> (20.25, -42.75)
  line L282 (20.25, -27.75) -> (9.75, -27.75)
  line L283 (9.75, -27.75) -> (9.75, -17.25)
  line L284 (9.75, -17.25) -> (20.25, -17.25)
  line L285 (20.25, -17.25) -> (20.25, -27.75)
  line L286 (20.25, -12.75) -> (9.75, -12.75)
  line L287 (9.75, -12.75) -> (9.75, -2.25)
  line L288 (9.75, -2.25) -> (20.25, -2.25)
  line L289 (20.25, -2.25) -> (20.25, -12.75)
  line L290 (20.25, 2.25) -> (9.75, 2.25)
  line L291 (9.75, 2.25) -> (9.75, 12.75)
  line L292 (9.75, 12.75) -> (20.25, 12.75)
  line L293 (20.25, 12.75) -> (20.25, 2.25)
  line L294 (20.25, 17.25) -> (9.75, 17.25)
  line L295 (9.75, 17.25) -> (9.75, 27.75)
  line L296 (9.75, 27.75) -> (20.25, 27.75)
  line L297 (20.25, 27.75) -> (20.25, 17.25)
  line L298 (20.25, 32.25) -> (9.75, 32.25)
  line L299 (9.75, 32.25) -> (9.75, 42.75)
  line L300 (9.75, 42.75) -> (20.25, 42.75)
  line L301 (20.25, 42.75) -> (20.25, 32.25)
  line L302 (20.25, 47.25) -> (9.75, 47.25)
  line L303 (9.75, 47.25) -> (9.75, 57.75)
  line L304 (9.75, 57.75) -> (20.25, 57.75)
  line L305 (20.25, 57.75) -> (20.25, 47.25)
  line L306 (20.25, 62.25) -> (9.75, 62.25)
  line L307 (9.75, 62.25) -> (9.75, 72.75)
  line L308 (9.75, 72.75) -> (20.25, 72.75)
  line L309 (20.25, 72.75) -> (20.25, 62.25)
  line L310 (20.25, 77.25) -> (9.75, 77.25)
  line L311 (9.75, 77.25) -> (9.75, 87.75)
  line L312 (9.75, 87.75) -> (20.25, 87.75)
  line L313 (20.25, 87.75) -> (20.25, 77.25)
  line L314 (20.25, 92.25) -> (9.75, 92.25)
  line L315 (9.75, 92.25) -> (9.75, 102.75)
  line L316 (9.75, 102.75) -> (20.25, 102.75)
  line L317 (20.25, 102.75) -> (20.25, 92.25)
  line L318 (20.25, 107.25) -> (9.75, 107.25)
  line L319 (9.75, 107.25) -> (9.75, 117.75)
  line L320 (9.75, 117.75) -> (20.25, 117.75)
  line L321 (20.25, 117.75) -> (20.25, 107.25)
  line L322 (35.25, -117.75) -> (24.75, -117.75)
  line L323 (24.75, -117.75) -> (24.75, -107.25)
  line L324 (24.75, -107.25) -> (35.25, -107.25)
  line L325 (35.25, -107.25) -> (35.25, -117.75)
  line L326 (35.25, -102.75) -> (24.75, -102.75)
  line L327 (24.75, -102.75) -> (24.75, -92.25)
  line L328 (24.75, -92.25) -> (35.25, -92.25)
  line L329 (35.25, -92.25) -> (35.25, -102.75)
  line L330 (35.25, -87.75) -> (24.75, -87.75)
  line L331 (24.75, -87.75) -> (24.75, -77.25)
  line L332 (24.75, -77.25) -> (35.25, -77.25)
  line L333 (35.25, -77.25) -> (35.25, -87.75)
  line L334 (35.25, -72.75) -> (24.75, -72.75)
  line L335 (24.75, -72.75) -> (24.75, -62.25)
  line L336 (24.75, -62.25) -> (35.25, -62.25)
  line L337 (35.25, -62.25) -> (35.25, -72.75)
  line L338 (35.25, -57.75) -> (24.75, -57.75)
  line L339 (24.75, -57.75) -> (24.75, -47.25)
  line L340 (24.75, -47.25) -> (35.25, -47.25)
  line L341 (35.25, -47.25) -> (35.25, -57.75)
  line L342 (35.25, -42.75) -> (24.75, -42.75)
  line L343 (24.75, -42.75) -> (24.75, -32.25)
  line L344 (24.75, -32.25) -> (35.25, -32.25)
  line L345 (35.25, -32.25) -> (35.25, -42.75)
  line L346 (35.25, -27.75) -> (24.75, -27.75)
  line L347 (24.75, -27.75) -> (24.75, -17.25)
  line L348 (24.75, -17.25) -> (35.25, -17.25)
  line L349 (35.25, -17.25) -> (35.25, -27.75)
  line L350 (35.25, -12.75) -> (24.75, -12.75)
  line L351 (24.75, -12.75) -> (24.75, -2.25)
  line L352 (24.75, -2.25) -> (35.25, -2.25)
  line L353 (35.25, -2.25) -> (35.25, -12.75)
  line L354 (35.25, 2.25) -> (24.75, 2.25)
  line L355 (24.75, 2.25) -> (24.75, 12.75)
  line L356 (24.75, 12.75) -> (35.25, 12.75)
  line L357 (35.25, 12.75) -> (35.25, 2.25)
  line L358 (35.25, 17.25) -> (24.75, 17.25)
  line L359 (24.75, 17.25) -> (24.75, 27.75)
  line L360 (24.75, 27.75) -> (35.25, 27.75)
  line L361 (35.25, 27.75) -> (35.25, 17.25)
  line L362 (35.25, 32.25) -> (24.75, 32.25)
  line L363 (24.75, 32.25) -> (24.75, 42.75)
  line L364 (24.75, 42.75) -> (35.25, 42.75)
  line L365 (35.25, 42.75) -> (35.25, 32.25)
  line L366 (35.25, 47.25) -> (24.75, 47.25)
  line L367 (24.75, 47.25) -> (24.75, 57.75)
  line L368 (24.75, 57.75) -> (35.25, 57.75)
  line L369 (35.25, 57.75) -> (35.25, 47.25)
  line L370 (35.25, 62.25) -> (24.75, 62.25)
  line L371 (24.75, 62.25) -> (24.75, 72.75)
  line L372 (24.75, 72.75) -> (35.25, 72.75)
  line L373 (35.25, 72.75) -> (35.25, 62.25)
  line L374 (35.25, 77.25) -> (24.75, 77.25)
  line L375 (24.75, 77.25) -> (24.75, 87.75)
  line L376 (24.75, 87.75) -> (35.25, 87.75)
  line L377 (35.25, 87.75) -> (35.25, 77.25)
  line L378 (35.25, 92.25) -> (24.75, 92.25)
  line L379 (24.75, 92.25) -> (24.75, 102.75)
  line L380 (24.75, 102.75) -> (35.25, 102.75)
  line L381 (35.25, 102.75) -> (35.25, 92.25)
  line L382 (35.25, 107.25) -> (24.75, 107.25)
  line L383 (24.75, 107.25) -> (24.75, 117.75)
  line L384 (24.75, 117.75) -> (35.25, 117.75)
  line L385 (35.25, 117.75) -> (35.25, 107.25)
  line L386 (50.25, -117.75) -> (39.75, -117.75)
  line L387 (39.75, -117.75) -> (39.75, -107.25)
  line L388 (39.75, -107.25) -> (50.25, -107.25)
  line L389 (50.25, -107.25) -> (50.25, -117.75)
  line L390 (50.25, -102.75) -> (39.75, -102.75)
  line L391 (39.75, -102.75) -> (39.75, -92.25)
  line L392 (39.75, -92.25) -> (50.25, -92.25)
  line L393 (50.25, -92.25) -> (50.25, -102.75)
  line L394 (50.25, -87.75) -> (39.75, -87.75)
  line L395 (39.75, -87.75) -> (39.75, -77.25)
  line L396 (39.75, -77.25) -> (50.25, -77.25)
  line L397 (50.25, -77.25) -> (50.25, -87.75)
  line L398 (50.25, -72.75) -> (39.75, -72.75)
  line L399 (39.75, -72.75) -> (39.75, -62.25)
  line L400 (39.75, -62.25) -> (50.25, -62.25)
  line L401 (50.25, -62.25) -> (50.25, -72.75)
  line L402 (50.25, -57.75) -> (39.75, -57.75)
  line L403 (39.75, -57.75) -> (39.75, -47.25)
  line L404 (39.75, -47.25) -> (50.25, -47.25)
  line L405 (50.25, -47.25) -> (50.25, -57.75)
  line L406 (50.25, -42.75) -> (39.75, -42.75)
  line L407 (39.75, -42.75) -> (39.75, -32.25)
  line L408 (39.75, -32.25) -> (50.25, -32.25)
  line L409 (50.25, -32.25) -> (50.25, -42.75)
  line L410 (50.25, -27.75) -> (39.75, -27.75)
  line L411 (39.75, -27.75) -> (39.75, -17.25)
  line L412 (39.75, -17.25) -> (50.25, -17.25)
  line L413 (50.25, -17.25) -> (50.25, -27.75)
  line L414 (50.25, -12.75) -> (39.75, -12.75)
  line L415 (39.75, -12.75) -> (39.75, -2.25)
  line L416 (39.75, -2.25) -> (50.25, -2.25)
  line L417 (50.25, -2.25) -> (50.25, -12.75)
  line L418 (50.25, 2.25) -> (39.75, 2.25)
  line L419 (39.75, 2.25) -> (39.75, 12.75)
  line L420 (39.75, 12.75) -> (50.25, 12.75)
  line L421 (50.25, 12.75) -> (50.25, 2.25)
  line L422 (50.25, 17.25) -> (39.75, 17.25)
  line L423 (39.75, 17.25) -> (39.75, 27.75)
  line L424 (39.75, 27.75) -> (50.25, 27.75)
  line L425 (50.25, 27.75) -> (50.25, 17.25)
  line L426 (50.25, 32.25) -> (39.75, 32.25)
  line L427 (39.75, 32.25) -> (39.75, 42.75)
  line L428 (39.75, 42.75) -> (50.25, 42.75)
  line L429 (50.25, 42.75) -> (50.25, 32.25)
  line L430 (50.25, 47.25) -> (39.75, 47.25)
  line L431 (39.75, 47.25) -> (39.75, 57.75)
  line L432 (39.75, 57.75) -> (50.25, 57.75)
  line L433 (50.25, 57.75) -> (50.25, 47.25)
  line L434 (50.25, 62.25) -> (39.75, 62.25)
  line L435 (39.75, 62.25) -> (39.75, 72.75)
  line L436 (39.75, 72.75) -> (50.25, 72.75)
  line L437 (50.25, 72.75) -> (50.25, 62.25)
  line L438 (50.25, 77.25) -> (39.75, 77.25)
  line L439 (39.75, 77.25) -> (39.75, 87.75)
  line L440 (39.75, 87.75) -> (50.25, 87.75)
  line L441 (50.25, 87.75) -> (50.25, 77.25)
  line L442 (50.25, 92.25) -> (39.75, 92.25)
  line L443 (39.75, 92.25) -> (39.75, 102.75)
  line L444 (39.75, 102.75) -> (50.25, 102.75)
  line L445 (50.25, 102.75) -> (50.25, 92.25)
  line L446 (50.25, 107.25) -> (39.75, 107.25)
  line L447 (39.75, 107.25) -> (39.75, 117.75)
  line L448 (39.75, 117.75) -> (50.25, 117.75)
  line L449 (50.25, 117.75) -> (50.25, 107.25)
  line L450 (24.75, -87.75) -> (50.25, -87.75)
  line L451 (50.25, -87.75) -> (50.25, -77.25)
  line L452 (50.25, -77.25) -> (24.75, -77.25)
  line L453 (24.75, -77.25) -> (24.75, -87.75)
  line L454 (24.75, -72.75) -> (50.25, -72.75)
  line L455 (50.25, -72.75) -> (50.25, -62.25)
  line L456 (50.25, -62.25) -> (24.75, -62.25)
  line L457 (24.75, -62.25) -> (24.75, -72.75)
  line L458 (24.75, -57.75) -> (50.25, -57.75)
  line L459 (50.25, -57.75) -> (50.25, -47.25)
  line L460 (50.25, -47.25) -> (24.75, -47.25)
  line L461 (24.75, -47.25) -> (24.75, -57.75)
  line L462 (24.75, -42.75) -> (50.25, -42.75)
  line L463 (50.25, -42.75) -> (50.25, -32.25)
  line L464 (50.25, -32.25) -> (24.75, -32.25)
  line L465 (24.75, -32.25) -> (24.75, -42.75)
  line L466 (24.75, -27.75) -> (50.25, -27.75)
  line L467 (50.25, -27.75) -> (50.25, -17.25)
  line L468 (50.25, -17.25) -> (24.75, -17.25)
  line L469 (24.75, -17.25) -> (24.75, -27.75)
  line L470 (24.75, -12.75) -> (50.25, -12.75)
  line L471 (50.25, -12.75) -> (50.25, -2.25)
  line L472 (50.25, -2.25) -> (24.75, -2.25)
  line L473 (24.75, -2.25) -> (24.75, -12.75)
  line L474 (24.75, 2.25) -> (50.25, 2.25)
  line L475 (50.25, 2.25) -> (50.25, 12.75)
  line L476 (50.25, 12.75) -> (24.75, 12.75)
  line L477 (24.75, 12.75) -> (24.75, 2.25)
  line L478 (24.75, 17.25) -> (50.25, 17.25)
  line L479 (50.25, 17.25) -> (50.25, 27.75)
  line L480 (50.25, 27.75) -> (24.75, 27.75)
  line L481 (24.75, 27.75) -> (24.75, 17.25)
  line L482 (24.75, 32.25) -> (50.25, 32.25)
  line L483 (50.25, 32.25) -> (50.25, 42.75)
  line L484 (50.25, 42.75) -> (24.75, 42.75)
  line L485 (24.75, 42.75) -> (24.75, 32.25)
  line L486 (24.75, 47.25) -> (50.25, 47.25)
  line L487 (50.25, 47.25) -> (50.25, 57.75)
  line L488 (50.25, 57.75) -> (24.75, 57.75)
  line L489 (24.75, 57.75) -> (24.75, 47.25)
  line L490 (24.75, 62.25) -> (50.25, 62.25)
  line L491 (50.25, 62.25) -> (50.25, 72.75)
  line L492 (50.25, 72.75) -> (24.75, 72.75)
  line L493 (24.75, 72.75) -> (24.75, 62.25)
  line L494 (24.75, 77.25) -> (50.25, 77.25)
  line L495 (50.25, 77.25) -> (50.25, 87.75)
  line L496 (50.25, 87.75) -> (24.75, 87.75)
  line L497 (24.75, 87.75) -> (24.75, 77.25)
  line L498 (24.75, 92.25) -> (50.25, 92.25)
  line L499 (50.25, 92.25) -> (50.25, 102.75)
  line L500 (50.25, 102.75) -> (24.75, 102.75)
  line L501 (24.75, 102.75) -> (24.75, 92.25)
  line L502 (24.75, 107.25) -> (50.25, 107.25)
  line L503 (50.25, 107.25) -> (50.25, 117.75)
  line L504 (50.25, 117.75) -> (24.75, 117.75)
  line L505 (24.75, 117.75) -> (24.75, 107.25)
  line L506 (9.75, -87.75) -> (20.25, -87.75)
  line L507 (20.25, -87.75) -> (20.25, -69.75)
  line L508 (20.25, -69.75) -> (9.75, -69.75)
  line L509 (9.75, -69.75) -> (9.75, -87.75)
  line L510 (9.75, -47.25) -> (20.25, -47.25)
  line L511 (20.25, -47.25) -> (20.25, -65.25)
  line L512 (20.25, -65.25) -> (9.75, -65.25)
  line L513 (9.75, -65.25) -> (9.75, -47.25)
  line L514 (9.75, -42.75) -> (20.25, -42.75)
  line L515 (20.25, -42.75) -> (20.25, -24.75)
  line L516 (20.25, -24.75) -> (9.75, -24.75)
  line L517 (9.75, -24.75) -> (9.75, -42.75)
  line L518 (9.75, -20.25) -> (20.25, -20.25)
  line L519 (20.25, -20.25) -> (20.25, -9.75)
  line L520 (20.25, -9.75) -> (9.75, -9.75)